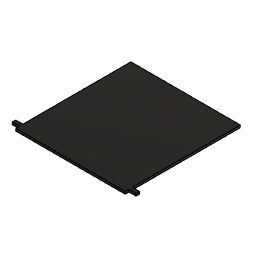
Flap v1 (Autodesk Fusion 360 design; units mm, degrees)
Autodesk Fusion 360 part; units mm, degrees
sketch "Sketch1" plane through (0, 0, 0) normal (0, 0, 1) x (1, 0, 0)
  line L0 (0, 0) -> (38, 0)
  line L1 (38, 40) -> (0, 40)
  line L2 (38, 2.5) -> (40.5, 2.5)
  line L3 (40.5, 2.5) -> (40.5, 1.3)
  line L4 (40.5, 1.3) -> (38, 1.3)
  line L5 (19, 40) -> (19, 0) construction
  line L6 (0, 2.5) -> (-2.5, 2.5)
  line L7 (-2.5, 2.5) -> (-2.5, 1.3)
  line L8 (-2.5, 1.3) -> (0, 1.3)
  line L9 (38, 0) -> (38, 1.3)
  line L10 (38, 2.5) -> (38, 40)
  line L11 (0, 40) -> (0, 2.5)
  line L12 (0, 1.3) -> (0, 0)
  dimension "d1" = 38
  dimension "d2" = 40
  dimension "d3" = 2.5
  dimension "d4" = 1.2
  dimension "d5" = 1.3
  dimension "d6" = 38
  constraint horizontal L0
  constraint vertical L9
  constraint horizontal L1
  constraint vertical L11
  constraint coincident L0.start L12.end
  constraint horizontal L2
  constraint vertical L3
  constraint horizontal L4
  constraint coincident L2.start L9
  constraint midpoint L1 L5.start
  constraint midpoint L0 L5.end
  constraint symmetric L2.start L5 L6.start
  constraint symmetric L2.end L5 L6.end
  constraint symmetric L3.end L5 L7.end
  constraint symmetric L4.end L5 L8.end
  measures "d1" distance of L0.start L0.end
  measures "d2" distance of L0.start L1.end
  measures "d3" distance of L2.start L2.end
  measures "d4" distance of L2.start L4.end
  measures "d5" distance of L0 L4
  measures "d6" distance of L1.start L1.end
extrude "Extrude1" add sketch "Sketch1" along normal blind 0.8 makes body 1
copy_body "Body->Comp1" bodies 1 removing the originals makes body 2 in component "Flap "
component "Flap " placed x (1, 0, 0) y (0, 1, 0) z (0, 0, 1) at (0, 0, 0)
named bodies: "Flap"
